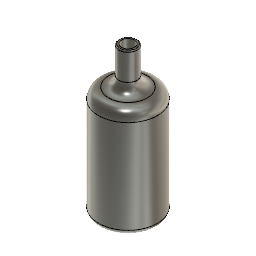
Semana2_Desafio4 v2 (Autodesk Fusion 360 design; units mm, degrees)
Autodesk Fusion 360 part; units mm, degrees
note: some values were not read from the file. Set by a fixed rule: which sketch regions a step uses.
sketch "Sketch3" plane through (0, 0, 0) normal (1, 0, 0) x (0, 1, 0)
  line L0 (0, 0) -> (28.7888, 0)
  line L1 (28.7888, 0) -> (28.7888, 106.2286)
  line L2 (28.7888, 106.2286) -> (8.923, 106.2286)
  line L3 (8.923, 106.2286) -> (8.923, 142.7466)
  line L4 (6.2937, 142.7466) -> (6.2937, 100.0936)
  line L5 (6.2937, 100.0936) -> (26.1595, 100.0936)
  line L6 (26.1595, 100.0936) -> (26.1595, 3.6859)
  line L7 (26.1595, 3.6859) -> (0, 3.6859)
  line L8 (0, 3.6859) -> (0, 0)
  line L9 (8.923, 142.7466) -> (6.2937, 142.7466)
  constraint coincident L0.start L8.end
  constraint horizontal L0
  constraint perpendicular L0 L1
  constraint perpendicular L1 L2
  constraint perpendicular L0 L3
  constraint perpendicular L4 L5
  constraint perpendicular L0 L6
  constraint perpendicular L6 L7
  constraint perpendicular L0 L8
  constraint vertical L4
  constraint perpendicular L4 L9
revolve "Revolve2" add sketch "Sketch3" angle 360 about axis through (0, 0, 1.75) along (0, 0, 1)
fillet "Fillet10" radius 10 1 edges at (-26.8406, 10.4105, 106.2286)
fillet "Fillet11" radius 10 1 edges at (-8.3191, 3.2267, 106.2286)
fillet "Fillet12" radius 1 1 edges at (-8.3191, 3.2267, 142.7466)
fillet "Fillet13" radius 5 1 edges at (-26.8406, 10.4105, 0)
